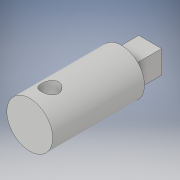
# Autodesk Inventor part: CrankP1_SBail
Saved by Autodesk Inventor 2019 (Build 230136000, 136)
## iProperties
Created: 2019-05-02
Part Number: CrankP1_SBail
Material: Generic
Document SubType Name: Modeling
Designer: samson.bailor
Density: 1 g/cm^3
Appearance: Default
Author: samson.bailor
Autodesk Inventor part; units mm, degrees
ref_plane "YZ Plane" through (0, 0, 0) normal (1, 0, 0) x (0, 1, 0)
ref_plane "XZ Plane" through (0, 0, 0) normal (0, 1, 0) x (-1, 0, 0)
ref_plane "XY Plane" through (0, 0, 0) normal (0, 0, 1) x (1, 0, 0)
sketch "Sketch1" plane through (0, 0, 0) normal (0, 0, 1) x (1, 0, 0)
  line L0 (-8.2623, 8.1273) -> (17.1377, 8.1273)
  line L1 (17.1377, 8.1273) -> (17.1377, -17.2727)
  line L2 (17.1377, -17.2727) -> (-8.2623, -17.2727)
  line L3 (-8.2623, -17.2727) -> (-8.2623, 8.1273)
  point P0 (0, 0)
  dimension "d0" = 25.4
  dimension "d1" = 25.4
  constraints: 8 end point, 2 parallel, 1 horizontal, 1 perpendicular
  measures "d0" distance of L1.end L2.end
  measures "d1" distance of L0.end L1.end
extrude "Extrusion1" add sketch "Sketch1" along normal blind 31.75
sketch "Sketch4" plane through (0, 0, 31.75) normal (0, 0, 1) x (1, 0, 0)
  line L0 (17.1377, 8.1273) -> (-8.2623, 8.1273) projected
  line L1 (4.4377, 8.1273) -> (4.4377, -17.2727)
  line L2 (-8.2623, -17.2727) -> (17.1377, -17.2727) projected
  circle A0 centre (4.4377, -4.5727) radius 25.4
  point P0 (0, 0)
  dimension "d11" = 50.8
  constraints: 3 midpoint, 2 end point, 1 centre point
  measures "d11" diameter of A0
extrude "Extrusion4" add sketch "Sketch4" along normal blind 101.6
sketch "Sketch5" plane through (-8.2623, 8.1273, 0) normal (0, 1, 0) x (1, 0, 0)
  line L0 (25.4, 0) -> (0, 0) projected
  line L1 (-12.7, -133.35) -> (38.1, -133.35) projected
  circle A0 centre (12.7, -111.125) radius 9.525
  point P0 (8.2623, 0)
  constraints: 1 centre point
extrude "Extrusion5" cut sketch "Sketch5" along normal blind 101.6
sketch "Sketch6" plane through (4.4377, 8.1273, 111.125) normal (0, 1, 0) x (1, 0, 0)
  circle A0 centre (0, 0) radius 9.525
  point P0 (-4.4377, 111.125)
  constraints: 1 centre point
extrude "Extrusion6" cut sketch "Sketch6" against normal blind 6.35
sketch "Sketch8" plane through (-8.2623, -17.2727, 0) normal (-1, 0, 0) x (0, 0, 1)
  line L0 (31.75, 25.4) -> (31.75, 0) projected
  line L1 (31.75, 12.7) -> (25.9588, 12.7)
  circle A0 centre (25.9588, 12.7) radius 3.175
  point P0 (0, 17.2727)
  dimension "d27" = 5.7912
  dimension "d28" = 6.35
  constraints: 2 end point, 1 centre point, 1 coincident, 1 horizontal, 1 midpoint
  measures "d27" distance of L1.start L1.end
  measures "d28" diameter of A0
extrude "Extrusion8" cut sketch "Sketch8" against normal blind 101.6
body "Solid1"
